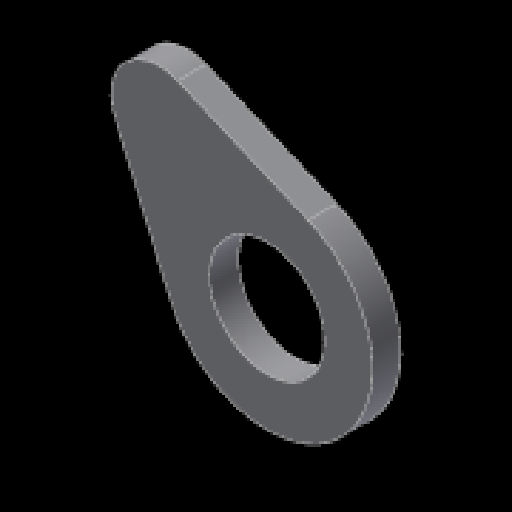
# Autodesk Inventor part: ChainTensionerMount
Saved by Autodesk Inventor 2025.2 (Build 292293000, 293)
## iProperties
Created: 2026-01-26
Part Number: ChainTensionerMount
Material: Generic
Document SubType Name: Sheet Metal
Designer: valer
Density: 1 g/cm^3
Sheet Metal Rule: Default_mm
Appearance: Default
Author: valer
Autodesk Inventor part; units mm, degrees
ref_plane "YZ Plane" through (0, 0, 0) normal (1, 0, 0) x (0, 1, 0)
ref_plane "XZ Plane" through (0, 0, 0) normal (0, 1, 0) x (-1, 0, 0)
ref_plane "XY Plane" through (0, 0, 0) normal (0, 0, 1) x (1, 0, 0)
sketch "ChainTensionerMount" plane through (0, 0, 0) normal (0, 0, 1) x (1, 0, 0)
  circle A0 centre (0, 0) radius 11
  circle A1 centre (-11.3137, 11.3137) radius 5
  line L0 (-9.362, 15.9171) -> (4.2937, 10.1274)
  line L1 (-15.9171, 9.362) -> (-10.1274, -4.2937)
  line L2 (-11.3137, 11.3137) -> (0, 0) construction
  line L3 (-22.8392, 0) -> (22.8392, 0) construction
  circle A2 centre (0, 0) radius 6
  circle A3 centre (-11.3137, 11.3137) radius 1.5
  circle A4 centre (-8.4853, 8.4853) radius 0.5
  line L4 (-7.7782, -7.7782) -> (7.7782, 7.7782) construction
  circle A5 centre (11.3137, -11.3137) radius 5
  line L5 (15.9171, -9.362) -> (10.1274, 4.2937)
  line L6 (9.362, -15.9171) -> (-4.2937, -10.1274)
  circle A6 centre (11.3137, -11.3137) radius 1.5
  point P0 (-4.2937, -10.1274)
  dimension "d0" = 22
  dimension "d1" = 10
  dimension "d2" = 45
  dimension "d3" = 12
  dimension "d5" = 3
  dimension "d6" = 1
  dimension "d7" = 12
  measures "d0" diameter of A0
  measures "d1" diameter of A1
  measures "d2" angle of L3 L2
  measures "d3" diameter of A2
  measures "d5" diameter of A3
  measures "d6" diameter of A4
  measures "d7" distance of point (0, 0) A4.centre
extrude "Plate1" add sketch "ChainTensionerMount" along normal blind 3
equation "\"d4\" = Thickness"
equation "\"BendRadius\" = Thickness"
equation "\"BendReliefWidth\" = Thickness"
equation "\"BendReliefDepth\" = 0.5 * Thickness"
equation "\"CornerReliefSize\" = 4 * Thickness"
equation "\"MinimumRemnant\" = 2 * Thickness"
equation "\"TransitionRadius\" = BendRadius"
equation "\"JacobiRadiusSize\" = BendRadius"
equation "\"GapSize\" = Thickness"
equation "\"Thickness\" = 3"
body "Solid1"
